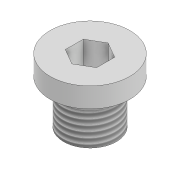
# Autodesk Inventor part: Tuerca_pieza_conectores
Saved by Autodesk Inventor 2022.3 (Build 263350000, 350)
## iProperties
Created: 2023-07-17
Part Number: Tuerca_pieza_conectores
Material: Genérico
Document SubType Name: Modeling
Designer: Usuario
Density: 1 g/cm^3
Appearance: Valor por defecto
Author: Usuario
Autodesk Inventor part; units mm, degrees
ref_plane "YZ Plane" through (0, 0, 0) normal (1, 0, 0) x (0, 1, 0)
ref_plane "XZ Plane" through (0, 0, 0) normal (0, 1, 0) x (-1, 0, 0)
ref_plane "XY Plane" through (0, 0, 0) normal (0, 0, 1) x (1, 0, 0)
sketch "Boceto1" plane through (0, 0, 0) normal (0, 1, 0) x (-1, 0, 0)
  circle A0 centre (0, 0) radius 7.275
  dimension "d0" = 14.55
  constraints: 1 centre point, 1 coincident
  measures "d0" diameter of A0
extrude "Extrusión1" add sketch "Boceto1" along normal blind 12
sketch "Boceto2" plane through (0, 12, 0) normal (0, 1, 0) x (1, 0, 0)
  circle A0 centre (0, 0) radius 11
  dimension "d3" = 22
  constraints: 1 centre point, 1 coincident
  measures "d3" diameter of A0
extrude "Extrusión2" add sketch "Boceto2" along normal blind 5.5
sketch "Boceto3" plane through (0, 17.5, 0) normal (0, 1, 0) x (1, 0, 0)
  line L0 (0, 0) -> (-4.325, 0)
  line L1 (-4.325, 2.497) -> (0, 4.9941)
  line L2 (0, 4.9941) -> (4.325, 2.497)
  line L3 (4.325, 2.497) -> (4.325, -2.497)
  line L4 (4.325, -2.497) -> (0, -4.9941)
  line L5 (0, -4.9941) -> (-4.325, -2.497)
  line L6 (-4.325, -2.497) -> (-4.325, 2.497)
  dimension "d6" = 4.325
  constraints: 14 end point, 1 coincident, 1 horizontal, 1 midpoint, 13 other
  measures "d6" distance of L0.start L0.end
extrude "Extrusión3" cut sketch "Boceto3" against normal blind 11.4
thread "Rosca1" size "M15x1.5" class "6g" standard "ANSI Metric M Profile" length 9
sketch "Boceto4" plane through (0, 12, 0) normal (0, -1, 0) x (1, 0, 0)
  circle A0 centre (0, 0) radius 7.275
  circle A1 centre (0, 0) radius 10
  dimension "d11" = 20
  constraints: 2 centre point, 2 coincident
  measures "d11" diameter of A1
extrude "Extrusión4" cut sketch "Boceto4" against normal blind 1
